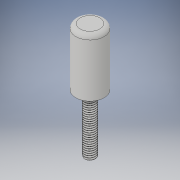
# Autodesk Inventor part: Battery Terminal
Saved by Autodesk Inventor 2017 (Build 210142000, 142)
## iProperties
Created: 2019-06-23
Part Number: Battery Terminal
Material: Generic
Document SubType Name: Modeling
Designer: Mitch
Density: 1 g/cm^3
Appearance: Default
Author: Mitch
Autodesk Inventor part; units mm, degrees
ref_plane "YZ Plane" through (0, 0, 0) normal (1, 0, 0) x (0, 1, 0)
ref_plane "XZ Plane" through (0, 0, 0) normal (0, 1, 0) x (-1, 0, 0)
ref_plane "XY Plane" through (0, 0, 0) normal (0, 0, 1) x (1, 0, 0)
sketch "Sketch1" plane through (0, 0, 0) normal (0, 1, 0) x (-1, 0, 0)
  circle A0 centre (0, 0) radius 3.9688
  dimension "d0" = 7.9375
  constraints: 1 centre point, 1 coincident
  measures "d0" diameter of A0
extrude "Extrusion1" add sketch "Sketch1" along normal blind 50.038
thread "Thread1" size "5/16-18 UNC" class "2A" standard "ANSI Unified Screw Threads" full length
sketch "Sketch3" plane through (0, 50.038, 0) normal (1, 0, 0) x (0, 0, 1)
  line L0 (3.9688, 0) -> (3.9688, 50.038)
  line L1 (3.9688, 50.038) -> (2.9225, 50.038)
  line L2 (2.9225, 50.038) -> (2.9225, 0)
  line L3 (2.9225, 0) -> (3.9688, 0)
  line L4 (0, -11.8541) -> (0, 60.3534) projected
  constraints: 8 end point
revolve "Revolution1" cut sketch "Sketch3" angle 360 about axis through (0, 50.038, 0) along (0, -1, 0)
sketch "Sketch4" plane through (0, 50.038, 0) normal (1, 0, 0) x (0, 0, 1)
  line L0 (3.9688, 0) -> (3.9688, 50.038)
  line L1 (3.9688, 50.038) -> (2.9225, 50.038)
  line L2 (2.9225, 50.038) -> (2.9225, 0)
  line L3 (2.9225, 0) -> (3.9688, 0)
  line L4 (0, -11.8541) -> (0, 60.3534) projected
  constraints: 8 end point
revolve "Revolution2" add sketch "Sketch4" angle 360 about axis through (0, 50.038, 0) along (0, -1, 0) separate body
sketch "Sketch2" plane through (0, 50.038, 0) normal (-1, 0, 0) x (0, -1, 0)
  line L0 (-0.8233, -2.994) -> (-0.7057, -2.994) construction
  line L1 (0.1175, -3.8976) -> (-0.0001, -4.1235) construction
  line L2 (-1.4112, -4.1235) -> (-1.5288, -3.8976) construction
  line L3 (-0.5881, -2.994) -> (-0.7057, -2.7681) construction
  line L4 (-0.7057, -2.7681) -> (-0.8233, -2.994) construction
  line L5 (-1.4112, -4.1235) -> (-1.2936, -3.8976) construction
  line L6 (-0.5881, -2.994) -> (-0.1177, -3.8976)
  line L7 (-1.5288, -3.8976) -> (-1.2936, -3.8976) construction
  arc A0 (-1.5288, -3.8976) -> (-1.4112, -3.9689) centre (-1.4112, -3.8363) ccw construction
  line L8 (0.1175, -3.8976) -> (-0.1177, -3.8976) construction
  line L9 (-1.4112, -4.1235) -> (-1.4112, -3.8976) construction
  line L10 (-0.0001, -4.1235) -> (-0.0001, -3.8976) construction
  line L11 (-0.7057, -2.7681) -> (-0.7057, -2.9226) construction
  line L12 (-1.4112, -3.9689) -> (-0.0001, -3.9689)
  arc A1 (-1.4112, -3.9689) -> (-1.2936, -3.8976) centre (-1.4112, -3.8363) ccw
  line L13 (-0.1177, -3.8976) -> (-0.0001, -4.1235) construction
  line L14 (-1.2936, -3.8976) -> (-0.8233, -2.994)
  line L15 (-0.0001, -0.0002) -> (-0.0001, 0.0177)
  line L16 (-0.0001, 0.0177) -> (-0.0001, -0.0002)
  line L17 (-0.0001, -0.0002) -> (0.0334, -0.0002)
  arc A2 (-0.1177, -3.8976) -> (-0.0001, -3.9689) centre (-0.0001, -3.8363) ccw
  arc A3 (-0.0001, -3.9689) -> (0.1175, -3.8976) centre (-0.0001, -3.8363) ccw construction
  arc A4 (-0.7057, -2.9226) -> (-0.8233, -2.994) centre (-0.7057, -3.0552) ccw
  arc A5 (-0.5881, -2.994) -> (-0.7057, -2.9226) centre (-0.7057, -3.0552) ccw
  line L18 (-0.7057, -2.9226) -> (-0.7057, -2.994) construction
  line L19 (-0.7057, -2.994) -> (-0.5881, -2.994) construction
  dimension "d5" = 55
  dimension "d6" = 0.2259
  dimension "d7" = 0.2259
  dimension "Sketch2_ThreadOffset" = 0
  dimension "Sketch2_MajorRadius" = 3.9688
  dimension "d10" = 1.4111
  dimension "Sketch2_MinorRadius" = 2.9225
  constraints: 40 end point, 12 point on circle, 10 parallel, 8 tangent, 6 centre point, 6 collinear, 2 midpoint, 2 point on line, 1 horizontal, 1 perpendicular, 3 other
  measures "d5" angle of L6 L14
  measures "d6" distance of L3.end L0.end
  measures "d7" distance of L1.end L10.end
  measures "Sketch2_ThreadOffset" distance between parallel lines of L15 L10
  measures "Sketch2_MajorRadius" distance from line of L12 L15.start
  measures "d10" distance from line of L1.end L9
  measures "Sketch2_MinorRadius" distance edge to line of A5 L17
coil "Coil1" sketch "Sketch2" operation cut axis through (0, 50.038, 0) along (0, -1, 0) pitch 1.4125 turns 37.422577 hand right bodies 2
sketch "Sketch5" plane through (0, 50.038, 0) normal (0, 1, 0) x (1, 0, 0)
  circle A0 centre (0, 0) radius 10.16
  dimension "d24" = 20.32
  constraints: 1 centre point, 1 coincident
  measures "d24" diameter of A0
extrude "Extrusion2" add sketch "Sketch5" against normal blind 8.8646 bodies 1
sketch "Sketch6" plane through (0, 50.038, 0) normal (0, 1, 0) x (1, 0, 0)
  circle A0 centre (0, 0) radius 10.16 projected
extrude "Extrusion3" add sketch "Sketch6" along normal blind 32.3088 bodies 1
fillet "Fillet1" radius 3.175 1 edges at (-10.16, 82.3468, 0)
equation "\"d5\" = d12"
equation "\"d6\" = 0.160083 * Sketch2_Pitch"
equation "\"d7\" = 0.160083 * Sketch2_Pitch"
equation "\"d10\" = Sketch2_Pitch"
equation "\"d12\" = 55deg"
equation "\"Sketch2_Pitch\" = 1.41111"
body "Solid1"
body "Solid2"
